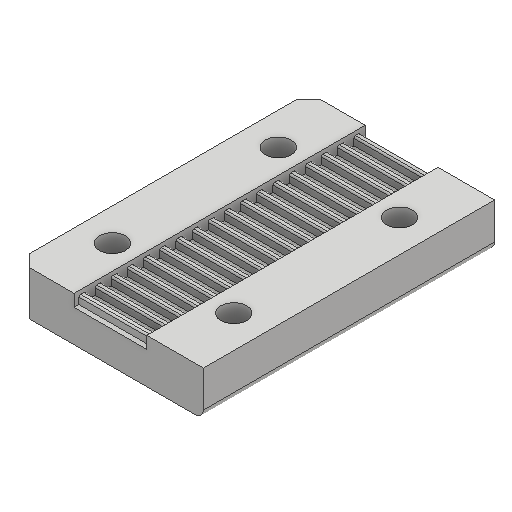
# Autodesk Inventor part: 3DP_ABS_Y_Axis_GT2_Belt_Clamp
Saved by Autodesk Inventor 2026.1 (Build 301233000, 233)
## iProperties
Created: 2016-06-19
Part Number: 3DP_ABS_Y_Axis_GT2_Belt_Clamp
Material: Ogólny
Document SubType Name: Modeling
Designer: Andrzej
Density: 1 g/cm^3
Appearance: Domyślna
Mass: 3.72076 g
Surface Area: 26.3708 cm^2
Volume: 3.72076 cm^3
Author: Andrzej
Autodesk Inventor part; units mm, degrees
ref_plane "YZ Plane" through (0, 0, 0) normal (1, 0, 0) x (0, 1, 0)
ref_plane "XZ Plane" through (0, 0, 0) normal (0, 1, 0) x (-1, 0, 0)
ref_plane "XY Plane" through (0, 0, 0) normal (0, 0, 1) x (1, 0, 0)
sketch "Szkic1" plane through (0, 0, 0) normal (0, 0, 1) x (1, 0, 0)
  line L0 (-12.5417, 6.9676) -> (10.4583, 6.9676)
  line L1 (10.4583, 6.9676) -> (10.4583, -29.0324)
  line L2 (10.4583, -29.0324) -> (-12.5417, -29.0324)
  line L3 (-12.5417, -29.0324) -> (-12.5417, 6.9676)
  point P0 (0, 0)
  dimension "d0" = 23
  dimension "d1" = 36
  constraints: 8 end point, 2 parallel, 1 horizontal, 1 perpendicular
  measures "d0" distance of L1.end L2.end
  measures "d1" distance of L0.end L1.end
extrude "Wyciągnięcie proste1" add sketch "Szkic1" along normal blind 4
fillet "Zaokrąglenie1" radius 1 1 edges at (10.4583, -11.0324, 0)
sketch "Szkic2" plane through (0, 0, 4) normal (0, 0, 1) x (1, 0, 0)
  line L0 (10.4583, 6.9676) -> (-12.5417, 6.9676) projected
  line L1 (-12.5417, 6.9676) -> (-12.5417, -29.0324) projected
  line L2 (-12.5417, -29.0324) -> (10.4583, -29.0324) projected
  line L3 (10.4583, -29.0324) -> (10.4583, 6.9676) projected
  line L4 (-5.5417, -29.0324) -> (-5.5417, 6.9676)
  line L5 (3.4583, -29.0324) -> (3.4583, 6.9676)
  point P0 (0, 0)
  dimension "d5" = 9
  dimension "d6" = 23
  dimension "d7" = 7
  constraints: 4 end point, 4 point on line, 2 perpendicular
  measures "d5" distance between parallel lines of L5 L4
  measures "d6" distance between parallel lines of L3 L1
  measures "d7" distance between parallel lines of L1 L4
extrude "Wyciągnięcie proste2" add sketch "Szkic2" along normal blind 1.5 contours L3 L2 L5 L0 | L4 L2 L1 L0
sketch "Szkic3" plane through (-5.5417, -29.0324, 4) normal (1, 0, 0) x (0, 0, -1)
  line L0 (4, 0) -> (4, 36) projected
  line L1 (4, 0) -> (-1.5, 0) projected
  line L2 (-1.5, 36) -> (-1.5, 0) projected
  line L3 (4, 36) -> (-1.5, 36) projected
  line L4 (-1, 0.6) -> (0, 0.6)
  line L5 (0, 0.6) -> (0, 1.4)
  line L6 (0, 1.4) -> (-1, 1.4)
  line L7 (-1, 1.4) -> (-1, 0.6)
  point P0 (4, 29.0324)
  dimension "d62" = 1
  dimension "d63" = 0.8
  dimension "d64" = 0.5
  dimension "d65" = 0.6
  constraints: 8 end point, 2 parallel, 1 horizontal, 1 perpendicular, 1 vertical
  measures "d62" distance of L6.end L5.end
  measures "d63" distance of L5.end L4.end
  measures "d64" distance between parallel lines of L2 L7
  measures "d65" distance between parallel lines of L1 L4
extrude "Wyciągnięcie proste3" add sketch "Szkic3" along normal blind 9 contours L7 L6 L5 L4
fillet "Zaokrąglenie2" radius 0.2 2 edges at (-1.0417, -28.4324, 5) (-1.0417, -27.6324, 5)
chamfer "Faza1" distance 1.5 angle 45 2 edges at (-12.5417, 6.9676, 2.75) (-12.5417, -29.0324, 2.75)
sketch "Szkic4" plane through (0, 0, 5.5) normal (0, 0, 1) x (1, 0, 0)
  line L0 (-11.0417, -29.0324) -> (-12.5417, -27.5324) projected
  line L1 (3.4583, -29.0324) -> (10.4583, -29.0324) projected
  line L2 (10.4583, -29.0324) -> (10.4583, 6.9676) projected
  line L3 (10.4583, 6.9676) -> (3.4583, 6.9676) projected
  line L4 (-5.5417, 6.9676) -> (-11.0417, 6.9676) projected
  line L5 (-12.5417, 5.4676) -> (-11.0417, 6.9676) projected
  line L6 (-12.5417, 5.4676) -> (-12.5417, -27.5324) projected
  line L7 (9.4583, -29.0324) -> (9.4583, 6.9676) projected
  line L8 (3.4583, 6.9676) -> (3.4583, -29.0324) projected
  line L9 (-11.0417, -29.0324) -> (-5.5417, -29.0324) projected
  line L10 (-5.5417, -29.0324) -> (-5.5417, 6.9676) projected
  point P0 (0, 0)
  point P1 (6.4583, -0.7824)
  point P2 (-8.5417, -0.7824)
  point P3 (-8.5417, -21.2824)
  point P4 (6.4583, -21.2824)
  dimension "d25" = 4
  dimension "d26" = 4
  dimension "d27" = 4
  dimension "d28" = 7.75
  dimension "d29" = 7.75
  dimension "d30" = 7.75
  dimension "d31" = 4
  dimension "d32" = 7.75
  measures "d25" distance from line of L2 point (6.458, -0.782)
  measures "d26" distance from line of point (-8.542, -0.782) L6
  measures "d27" distance from line of L6 point (-8.542, -21.282)
  measures "d28" distance from line of L3 point (6.458, -0.782)
  measures "d29" distance from line of L4 point (-8.542, -0.782)
  measures "d30" distance from line of L1 point (-8.542, -21.282)
  measures "d31" distance from line of L2 point (6.458, -21.282)
  measures "d32" distance from line of L1 point (6.458, -21.282)
hole "Otwór1" at (6.4583, -0.7824, 5.5) at (-8.5417, -0.7824, 5.5) at (-8.5417, -21.2824, 5.5) at (6.4583, -21.2824, 5.5) direction (0, 0, -1) diameter 3.2 end through all
pattern_linear "Szyk prostokątny1" count 18 spacing 2 along (0, 1, 0) of "Wyciągnięcie proste3", "Zaokrąglenie2"
equation "\"d7\" = -0.5 * d5 + 0.5 * d6"
equation "\"d26\" = d25"
equation "\"d27\" = d25"
equation "\"d29\" = d28"
equation "\"d30\" = d28"
